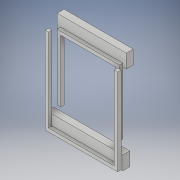
# Autodesk Inventor part: Foldedcapballliftholders
Saved by Autodesk Inventor 2017 (Build 210142000, 142)
## iProperties
Created: 2017-05-27
Part Number: Foldedcapballliftholders
Material: Generic
Document SubType Name: Modeling
Designer: User
Density: 1 g/cm^3
Appearance: Default
Author: User
Autodesk Inventor part; units mm, degrees
ref_plane "YZ Plane" through (0, 0, 0) normal (1, 0, 0) x (0, 1, 0)
ref_plane "XZ Plane" through (0, 0, 0) normal (0, 1, 0) x (-1, 0, 0)
ref_plane "XY Plane" through (0, 0, 0) normal (0, 0, 1) x (1, 0, 0)
sketch "Sketch1" plane through (0, 0, 0) normal (0, 0, 1) x (1, 0, 0)
  line L0 (0, 0) -> (254, 0)
  line L1 (254, 0) -> (254, 50.8)
  line L2 (254, 50.8) -> (0, 50.8)
  line L3 (0, 50.8) -> (0, 0)
  dimension "d0" = 254
  dimension "d1" = 50.8
  constraints: 8 end point, 2 parallel, 1 horizontal, 1 perpendicular
  measures "d0" distance of L2.end L1.end
  measures "d1" distance between parallel lines of L0 L2
extrude "Extrusion1" add sketch "Sketch1" along normal blind 25.4
sketch "Sketch2" plane through (0, 0, 25.4) normal (0, 0, 1) x (1, 0, 0)
  line L0 (0, 0) -> (254, 0) projected
  line L1 (0, 50.8) -> (0, 0) projected
  line L2 (0, -254) -> (254, -254)
  line L3 (254, -254) -> (254, -304.8)
  line L4 (254, -304.8) -> (0, -304.8)
  line L5 (0, -304.8) -> (0, -254)
  dimension "d4" = 254
  dimension "d5" = 0
  dimension "d6" = 50.8
  constraints: 8 end point, 2 parallel, 1 horizontal, 1 perpendicular
  measures "d4" distance from line of L0 L2.start
  measures "d5" distance from line of L2.start L1
  measures "d6" distance of L2.end L3.end
extrude "Extrusion2" add sketch "Sketch2" along normal blind 25.4
sketch "Sketch3" plane through (0, 0, 25.4) normal (0, 0, 1) x (1, 0, 0)
  line L0 (0, 0) -> (254, 0) projected
  line L1 (12.7, 0) -> (241.3, 0)
  line L2 (241.3, 0) -> (241.3, 12.7)
  line L3 (241.3, 12.7) -> (12.7, 12.7)
  line L4 (12.7, 12.7) -> (12.7, 0)
  dimension "d9" = 12.7
  constraints: 8 end point, 2 parallel, 1 horizontal, 1 perpendicular, 1 point on line
  measures "d9" distance of L2.end L1.end
extrude "Extrusion3" add sketch "Sketch3" along normal blind 12.7
thicken "Thicken1" operation add thickness 12.7 both sides no extend neighbours yes toward (1, 0, 0) faces at (254, -270.9333, 33.8667)
thicken "Thicken2" operation add thickness 12.7 both sides no extend neighbours yes toward (-1, 0, 0) faces at (0, -287.8667, 33.8667)
sketch "Sketch4" plane through (0, 0, 50.8) normal (0, 0, 1) x (1, 0, 0)
  point P0 (0, 0)
sketch "Sketch5" plane through (0, 0, 50.8) normal (0, 0, 1) x (1, 0, 0)
  point P0 (0, 0)
sketch "Sketch6" plane through (0, 0, 50.8) normal (0, 0, 1) x (1, 0, 0)
  point P0 (0, 0)
sketch "Sketch7" plane through (0, 0, 50.8) normal (0, 0, 1) x (1, 0, 0)
  line L0 (-12.7, -304.8) -> (266.7, -304.8) projected
  line L1 (-6.35, -304.8) -> (260.35, -304.8)
  line L2 (260.35, -304.8) -> (260.35, -292.1)
  line L3 (260.35, -292.1) -> (-6.35, -292.1)
  line L4 (-6.35, -292.1) -> (-6.35, -304.8)
  point P0 (0, 0)
  dimension "d16" = 12.7
  constraints: 8 end point, 2 parallel, 2 point on line, 1 horizontal, 1 perpendicular
  measures "d16" distance of L2.end L1.end
extrude "Extrusion4" add sketch "Sketch7" along normal blind 12.7
sketch "Sketch8" plane through (-6.35, -292.1, 50.8) normal (0, 1, 0) x (1, 0, 0)
  line L0 (0, 0) -> (0, -12.7) projected
  line L1 (0, 0) -> (266.7, 0) projected
  line L2 (0, -12.7) -> (12.7, -12.7)
  line L3 (12.7, -12.7) -> (12.7, 0)
  line L4 (12.7, 0) -> (0, 0)
  line L5 (0, 0) -> (0, -12.7)
  line L6 (266.7, 0) -> (266.7, -12.7) projected
  line L7 (266.7, -12.7) -> (254, -12.7)
  line L8 (254, -12.7) -> (254, 0)
  line L9 (254, 0) -> (266.7, 0)
  line L10 (266.7, 0) -> (266.7, -12.7)
  point P0 (6.35, 50.8)
  dimension "d19" = 12.7
  dimension "d20" = 12.7
  constraints: 16 end point, 4 parallel, 2 horizontal, 2 perpendicular, 2 point on line
  measures "d19" distance of L4.end L3.end
  measures "d20" distance of L8.end L9.end
extrude "Extrusion5" add sketch "Sketch8" along normal blind 304.8
sketch "Sketch9" plane through (0, 0, 0) normal (0, -1, 0) x (1, 0, 0)
  line L0 (0, 25.4) -> (12.7, 25.4) projected
  line L1 (241.3, 38.1) -> (12.7, 38.1) projected
  line L2 (12.7, 25.4) -> (25.4, 25.4)
  line L3 (25.4, 25.4) -> (25.4, 38.1)
  line L4 (25.4, 38.1) -> (12.7, 38.1)
  line L5 (12.7, 38.1) -> (12.7, 25.4)
  line L6 (241.3, 25.4) -> (241.3, 38.1) projected
  line L7 (241.3, 38.1) -> (228.6, 38.1)
  line L8 (228.6, 38.1) -> (228.6, 25.4)
  line L9 (228.6, 25.4) -> (241.3, 25.4)
  line L10 (241.3, 25.4) -> (241.3, 38.1)
  point P0 (0, 0)
  dimension "d23" = 12.7
  dimension "d24" = 12.7
  dimension "d25" = 12.7
  constraints: 16 end point, 4 parallel, 2 horizontal, 2 perpendicular, 1 point on line
  measures "d23" distance of L4.end L3.end
  measures "d24" distance of L9.end L8.end
  measures "d25" distance of L8.end L7.end
extrude "Extrusion6" add sketch "Sketch9" along normal blind 228.6
body "Solid1"
